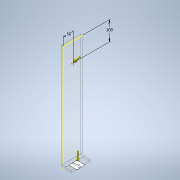
# Autodesk Inventor part: fea_leg
Saved by Autodesk Inventor 2020 (Build 240168000, 168)
## iProperties
Created: 2020-07-14
Part Number: fea_leg
Material: PMMA Plastic
Document SubType Name: Modeling
Designer: lu0248
Density: 1.188 g/cm^3
Appearance: Polycarbonate - Clear
Author: lu0248
Autodesk Inventor part; units mm, degrees
ref_plane "YZ Plane" through (0, 0, 0) normal (1, 0, 0) x (0, 1, 0)
ref_plane "XZ Plane" through (0, 0, 0) normal (0, 1, 0) x (-1, 0, 0)
ref_plane "XY Plane" through (0, 0, 0) normal (0, 0, 1) x (1, 0, 0)
sketch "Sketch1" plane through (0, 0, 0) normal (0, 0, 1) x (1, 0, 0)
  line L0 (0, 550) -> (0, 0)
  line L1 (0, 0) -> (50, 0)
  line L2 (50, 0) -> (50, 10)
  line L3 (50, 10) -> (10, 10)
  line L4 (10, 10) -> (10, 550)
  line L5 (10, 550) -> (0, 550)
  dimension "d1" = 550
  dimension "d2" = 50
  dimension "d3" = 10
  dimension "d4" = 10
  constraints: 12 end point, 5 perpendicular, 1 vertical
  measures "d1" distance between parallel lines of L1 L5
  measures "d2" distance between parallel lines of L0 L2
  measures "d3" distance between parallel lines of L1 L3
  measures "d4" distance between parallel lines of L0 L4
extrude "Extrusion1" add sketch "Sketch1" against normal blind 100
fillet "Fillet1" radius 10 2 edges at (10, 10, -50) (0, 0, -50)
sketch "Sketch2" plane through (10, 550, 0) normal (1, 0, 0) x (0, 0, -1)
  line L0 (0, -530) -> (0, 0) projected
  line L1 (0, 0) -> (100, 0) projected
  point P0 (0, -550)
  point P1 (50, -100)
  dimension "d8" = 50
  dimension "d9" = 100
  measures "d8" distance from line of L0 point (50, -100)
  measures "d9" distance from line of L1 point (50, -100)
body "Solid1"
